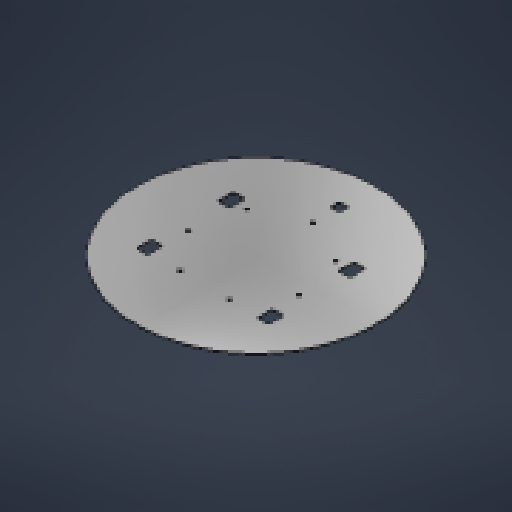
# Autodesk Inventor part: PLATE,SKIRT
Saved by Autodesk Inventor 2026.1 (Build 301233020, 233B)
## iProperties
Created: 2026-02-10
Part Number: PLATE,SKIRT
Material: Aluminum 6061
Document SubType Name: Sheet Metal
Designer: Owen L
Mass: 365.726 g
Surface Area: 1814.37 cm^2
Volume: 135.454 cm^3
Density: 2.7 g/cm^3
Sheet Metal Rule: Default
Appearance: Aluminum - Flat
Author: Owen L
Autodesk Inventor part; units mm, degrees
ref_plane "YZ Plane" through (0, 0, 0) normal (1, 0, 0) x (0, 1, 0)
ref_plane "XZ Plane" through (0, 0, 0) normal (0, 1, 0) x (-1, 0, 0)
ref_plane "XY Plane" through (0, 0, 0) normal (0, 0, 1) x (1, 0, 0)
sketch "Sketch1" plane through (0, 0, 0) normal (0, 1, 0) x (-1, 0, 0)
  line L0 (-105.7173, 121.3104) -> (105.7173, 121.3104) construction
  line L1 (105.7173, 121.3104) -> (105.7173, -121.3104) construction
  line L2 (105.7173, -121.3104) -> (-105.7173, -121.3104) construction
  line L3 (-105.7173, -121.3104) -> (-105.7173, 121.3104) construction
  line L4 (-105.7173, 121.3104) -> (105.7173, -121.3104) construction
  line L5 (105.7173, 121.3104) -> (-105.7173, -121.3104) construction
  circle A0 centre (0, 19.4053) radius 190.5
  line L6 (105.7173, 105.4354) -> (86.6673, 105.4354)
  line L7 (86.6673, 105.4354) -> (86.6673, 80.0354)
  line L8 (86.6673, 80.0354) -> (105.7173, 80.0354)
  line L9 (105.7173, 80.0354) -> (105.7173, 105.4354)
  line L10 (105.7173, -50.1396) -> (86.6673, -50.1396)
  line L11 (86.6673, -50.1396) -> (86.6673, -24.7396)
  line L12 (86.6673, -24.7396) -> (105.7173, -24.7396)
  line L13 (105.7173, -24.7396) -> (105.7173, -50.1396)
  line L14 (-7.9375, -105.4354) -> (-7.9375, -121.3104)
  line L15 (-7.9375, -121.3104) -> (7.9375, -121.3104)
  line L16 (7.9375, -121.3104) -> (7.9375, -105.4354)
  line L17 (7.9375, -105.4354) -> (-7.9375, -105.4354)
  line L18 (-7.9375, -105.4354) -> (7.9375, -121.3104) construction
  line L19 (-7.9375, -121.3104) -> (7.9375, -105.4354) construction
  line L20 (0, -247.2947) -> (0, 286.1053) construction
  line L21 (-105.7173, 105.4354) -> (-86.6673, 105.4354)
  line L22 (-86.6673, 105.4354) -> (-86.6673, 80.0354)
  line L23 (-86.6673, 80.0354) -> (-105.7173, 80.0354)
  line L24 (-105.7173, -50.1396) -> (-86.6673, -50.1396)
  line L25 (-86.6673, -50.1396) -> (-86.6673, -24.7396)
  line L26 (-86.6673, -24.7396) -> (-105.7173, -24.7396)
  line L27 (-105.7173, -50.1396) -> (-105.7173, -24.7396)
  line L28 (-105.7173, 80.0354) -> (-105.7173, 105.4354)
  line L29 (-61.595, -92.7354) -> (-29.845, -92.7354)
  line L30 (-29.845, -92.7354) -> (-29.845, -41.9354)
  line L31 (-29.845, -41.9354) -> (-61.595, -41.9354)
  line L32 (-61.595, -41.9354) -> (-61.595, -92.7354)
  line L33 (-61.595, -92.7354) -> (-29.845, -41.9354) construction
  line L34 (-29.845, -92.7354) -> (-61.595, -41.9354) construction
  line L35 (29.845, -92.7354) -> (61.595, -92.7354)
  line L36 (61.595, -92.7354) -> (61.595, -41.9354)
  line L37 (61.595, -41.9354) -> (29.845, -41.9354)
  line L38 (29.845, -41.9354) -> (29.845, -92.7354)
  line L39 (29.845, -92.7354) -> (61.595, -41.9354) construction
  line L40 (61.595, -92.7354) -> (29.845, -41.9354) construction
  circle A1 centre (0, 19.4053) radius 79.375
  point P0 (0, 0)
  point P1 (0, -71.0822)
  point P2 (70.746, -37.0127)
  point P3 (88.2188, 39.5407)
  point P4 (39.2611, 100.9318)
  point P5 (-39.2611, 100.9318)
  point P6 (-88.2188, 39.5407)
  point P7 (-70.746, -37.0127)
  point P8 (0, -113.3729)
  point P9 (-45.72, -67.3354)
  point P10 (45.72, -67.3354)
  point P11 (50.3756, -41.9354)
  point P12 (-50.3756, -41.9354)
  point P13 (-29.845, -54.1451)
  point P14 (29.845, -54.1451)
  point P15 (-94.6048, -108.6104)
  point P16 (94.6048, -108.6104)
  point P17 (94.6048, 111.7854)
  point P18 (-94.6048, 111.7854)
  dimension "d0" = 242.6208
  dimension "d1" = 211.4347
  dimension "d2" = 381
  dimension "d3" = 101.9051
  dimension "d4" = 90.4875
  dimension "d7" = 360
  dimension "d9" = 15.875
  dimension "d10" = 19.05
  dimension "d11" = 25.4
  dimension "d12" = 71.1708
  dimension "d13" = 15.875
  dimension "d29" = 158.75
  dimension "d30" = 53.975
  dimension "d31" = 45.72
  dimension "d32" = 50.8
  dimension "d33" = 31.75
  dimension "d34" = 9.525
  dimension "d35" = 11.1125
  dimension "d36" = 12.7
  constraints: 80 end point, 12 parallel, 11 symmetric about line, 8 midpoint, 6 perpendicular, 5 equal length, 5 horizontal, 5 vertical alignment, 3 collinear, 2 centre point, 2 horizontal alignment, 2 point on line, 1 coincident, 8 other
  measures "d0" distance of L0.end L1.end
  measures "d1" distance of L0.start L0.end
  measures "d2" diameter of A0
  measures "d3" distance from line of L0 A0.centre
  measures "d4" distance of A0.centre point (0, -71.082)
  measures "d9" distance between parallel lines of L6 L0
  measures "d10" distance of L6.start L6.end
  measures "d11" distance between parallel lines of L8 L6
  measures "d12" distance between parallel lines of L2 L10
  measures "d13" distance between parallel lines of L15 L17
  measures "d29" diameter of A1
  measures "d30" distance from line of L2 point (-45.72, -67.335)
  measures "d31" distance from line of L20 point (-45.72, -67.335)
  measures "d32" distance between parallel lines of L31 L29
  measures "d33" distance between parallel lines of L30 L32
  measures "d34" distance from line of L0 point (-94.605, 111.785)
  measures "d35" distance from line of L3 point (-94.605, 111.785)
  measures "d36" distance from line of L2 point (-94.605, -108.61)
extrude "Plate1" add sketch "Sketch1" along normal blind 1.524 contours A0 | L9 L8 L7 L6 | L10 L11 L12 L13 | L17 L16 L15 L14 | L21 L22 L23 L28 | L27 L26 L25 L24 | L32 L31 A1 L30 L29 | A1 L31 L30 | L30 L31 A1 L37 L38 | A1 L37 L36 L35 L38 | L38 L37 A1
extrude "Cut1" cut sketch "Sketch1" along normal blind 1.524 contours L9 L8 L7 L6 | L10 L11 L12 L13 | L17 L16 L15 L14 | L21 L22 L23 L28 | L27 L26 L25 L24 | L32 L31 A1 L30 L29 | A1 L31 L30 | L30 L31 A1 L37 L38 | A1 L37 L36 L35 L38 | L38 L37 A1
hole "Hole1" at (0, 0, -71.0822) at (-70.746, 0, -37.0127) at (-88.2188, 0, 39.5407) at (-39.2611, 0, 100.9318) at (39.2611, 0, 100.9318) at (88.2188, 0, 39.5407) at (70.746, 0, -37.0127) direction (0, 1, 0) diameter 6.35 depth 1.524 tip angle 118
fillet "Corner Round1" radius 3.175 30 edges at (86.6673, 0.762, -50.1396) (86.6673, 0.762, -24.7396) (105.7173, 0.762, -24.7396) (105.7173, 0.762, -50.1396) (7.9375, 0.762, -105.4354) (7.9375, 0.762, -121.3104) (-7.9375, 0.762, -105.4354) (-7.9375, 0.762, -121.3104) (-86.6673, 0.762, -24.7396) (-105.7173, 0.762, -24.7396) (86.6673, 0.762, 80.0354) (86.6673, 0.762, 105.4354) (105.7173, 0.762, 105.4354) (105.7173, 0.762, 80.0354) (-86.6673, 0.762, 80.0354) (-105.7173, 0.762, 80.0354) (-105.7173, 0.762, 105.4354) (-86.6673, 0.762, 105.4354) (-86.6673, 0.762, -50.1396) (-105.7173, 0.762, -50.1396) (50.3756, 0.762, -41.9354) (61.595, 0.762, -92.7354) (29.845, 0.762, -92.7354) (29.845, 0.762, -54.1451) (61.595, 0.762, -41.9354) (-29.845, 0.762, -54.1451) (-50.3756, 0.762, -41.9354) (-61.595, 0.762, -41.9354) (-29.845, 0.762, -92.7354) (-61.595, 0.762, -92.7354)
hole "Hole2" at (94.6048, 0, -108.6104) at (-94.6048, 0, -108.6104) at (-94.6048, 0, 111.7854) at (94.6048, 0, 111.7854) direction (0, 1, 0) diameter 4.9784 depth 1.524 tip angle 118 clearance for "Flat Head Machine Screw (82)" size "#10" standard "Ansi Unified Screw Threads"
equation "\"d19\" = Thickness"
equation "\"d26\" = Thickness"
equation "\"d42\" = Thickness"
equation "\"d18\" = Thickness"
equation "\"BendRadius\" = Thickness"
equation "\"BendReliefWidth\" = Thickness"
equation "\"BendReliefDepth\" = 0.5 * Thickness"
equation "\"CornerReliefSize\" = 4 * Thickness"
equation "\"MinimumRemnant\" = 2 * Thickness"
equation "\"TransitionRadius\" = BendRadius"
equation "\"JacobiRadiusSize\" = BendRadius"
equation "\"GapSize\" = Thickness"
equation "\"Thickness\" = 1.524"
body "Solid1"
